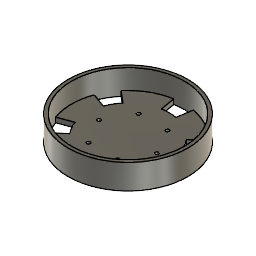
Drill guide FFBeast (Autodesk Fusion 360 design; units mm, degrees)
Autodesk Fusion 360 part; units mm, degrees
sketch "Sketch1" plane through (0, 0, 0) normal (0, 0, 1) x (1, 0, 0)
  circle A0 centre (0, 0) radius 68.25
  circle A1 centre (0, 0) radius 72.25
  line L0 (0, 0) -> (35, 0)
  circle A2 centre (35, 0) radius 2.1
  circle A3 centre (17.5, 30.3109) radius 2.1
  circle A4 centre (-17.5, 30.3109) radius 2.1
  circle A5 centre (-35, 0) radius 2.1
  circle A6 centre (-17.5, -30.3109) radius 2.1
  circle A7 centre (17.5, -30.3109) radius 2.1
  line L1 (0, 0) -> (3, 0)
  line L2 (0, 0) -> (68.25, 0)
  line L3 (0, 0) -> (64.134, 23.3429)
  line L4 (0, 0) -> (52.2825, 43.8703)
  line L5 (0, 0) -> (34.125, 59.1062)
  line L6 (0, 0) -> (11.8515, 67.2131)
  line L7 (0, 0) -> (-11.8515, 67.2131)
  line L8 (0, 0) -> (-34.125, 59.1062)
  line L9 (0, 0) -> (-52.2825, 43.8703)
  line L10 (0, 0) -> (-64.134, 23.3429)
  line L11 (0, 0) -> (-68.25, 0)
  line L12 (0, 0) -> (-64.134, -23.3429)
  line L13 (0, 0) -> (-52.2825, -43.8703)
  line L14 (0, 0) -> (-34.125, -59.1062)
  line L15 (0, 0) -> (-11.8515, -67.2131)
  line L16 (0, 0) -> (11.8515, -67.2131)
  line L17 (0, 0) -> (34.125, -59.1062)
  line L18 (0, 0) -> (52.2825, -43.8703)
  line L19 (0, 0) -> (64.134, -23.3429)
  circle A8 centre (0, 0) radius 50
  dimension "d1" = 136.5
  dimension "d2" = 4
  dimension "d3" = 35
  dimension "d4" = 4.2
  dimension "d6" = 360
  dimension "d12" = 360
  dimension "d13" = 100
  constraint coincident A0.centre A1.centre
  constraint horizontal L0
  constraint coincident L0.end A2.centre
  constraint coincident L0 L1.end
  constraint coincident A0 L2.end
  constraint parallel L0 L2
  measures "d1" diameter of A0
  measures "d3" distance of A0.centre L0.end
  measures "d4" diameter of A2
  measures "d13" diameter of A8
extrude "Extrude1" add sketch "Sketch1" along normal blind 6 contours A0 L2 L3 A8 | A0 L2 L19 A8 | L0 A2 L1 L2 L19 A8 | L0 A2 L1 L2 L3 A8 | A0 L4 L5 A8 | L3 L4 A8 | A0 L17 L18 A8 | L18 L19 A8 | A0 L5 L6 A8 | A3 L4 L5 A8 | A3 L5 L6 A8 | L6 L7 A8 | A4 L7 L8 A8 | A4 L8 L9 A8 | L9 L10 A8 | A5 L10 L11 A8 | A5 L11 L12 A8 | L12 L13 A8 | A6 L13 L14 A8 | A6 L14 L15 A8 | L15 L16 A8 | A7 L16 L17 A8 | A7 L17 L18 A8 | A0 L16 L17 A8 | A0 L7 L8 A8 | A0 L8 L9 A8 | A0 L10 L11 A8 | A0 L11 L12 A8 | A0 L13 L14 A8 | A0 L14 L15 A8
extrude "Extrude2" add sketch "Sketch1" along normal blind 30
